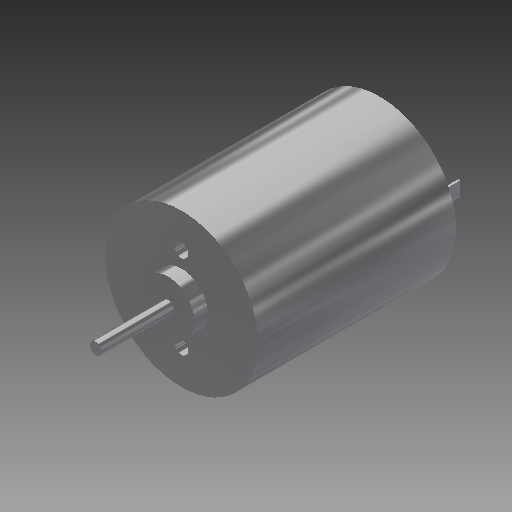
# Autodesk Inventor part: モーター(形だけ)
Saved by Autodesk Inventor 2019 (Build 230136000, 136)
## iProperties
Created: 2016-02-14
Part Number: モーター(形だけ)
Material: 一般
Document SubType Name: Modeling
Designer: 大空
Density: 2.93121 g/cm^3
Appearance: つや出し - 細かい格子状ナーリング
Mass: 75 g
Surface Area: 54.4313 cm^2
Volume: 25.5867 cm^3
Author: 大空
Autodesk Inventor part; units mm, degrees
ref_plane "YZ Plane" through (0, 0, 0) normal (1, 0, 0) x (0, 1, 0)
ref_plane "XZ Plane" through (0, 0, 0) normal (0, 1, 0) x (-1, 0, 0)
ref_plane "XY Plane" through (0, 0, 0) normal (0, 0, 1) x (1, 0, 0)
sketch "スケッチ1" plane through (0, 0, 0) normal (0, 0, 1) x (1, 0, 0)
  circle A0 centre (0, 0) radius 14.6
  circle A1 centre (0, 0) radius 5.025
  line L0 (0, 0) -> (8, 0)
  line L1 (0, 0) -> (-8, 0)
  circle A2 centre (0, 0) radius 1.15
  line L2 (-8, 0) -> (-8, -1.4)
  line L3 (-8, -1.4) -> (-8, 1.4)
  line L4 (8, 0) -> (8, -1.4)
  line L5 (8, -1.4) -> (8, 1.4)
  line L6 (8.4, -1.4) -> (8.4, 1.4)
  line L7 (-8.4, 1.4) -> (-8.4, -1.4)
  line L8 (-8.4, -1.4) -> (-8, -1.4)
  line L9 (-8.4, 1.4) -> (-8, 1.4)
  line L10 (8, -1.4) -> (8.4, -1.4)
  line L11 (8, 1.4) -> (8.4, 1.4)
  dimension "d0" = 29.2
  dimension "d1" = 10.05
  dimension "d2" = 8
  dimension "d3" = 8
  dimension "d6" = 2.3
  dimension "d21" = 1.4
  dimension "d22" = 2.8
  dimension "d23" = 1.4
  dimension "d24" = 2.8
  dimension "d25" = 0.4
  dimension "d26" = 0.4
  constraints: 24 end point, 4 vertical, 3 centre point, 3 coincident, 3 horizontal, 3 parallel, 2 point on line
  measures "d0" diameter of A0
  measures "d1" diameter of A1
  measures "d2" distance of L0.start L0.end
  measures "d3" distance of L0.start L1.end
  measures "d6" diameter of A2
  measures "d21" distance of L1.end L2.end
  measures "d22" distance of L2.end L3.end
  measures "d23" distance of L0.end L4.end
  measures "d24" distance of L4.end L5.end
  measures "d25" distance between parallel lines of L6 L4
  measures "d26" distance of L7.start L3.end
extrude "押し出し1" add sketch "スケッチ1" along normal blind 37.8 contours A0 | L0 A2 L1 A1 | L2 L8 L7 L9 L3 | A1 L1 A2 L0 | L5 L11 L6 L10 L4 | A2 L1 L0 | L0 L1 A2
extrude "押し出し2" add sketch "スケッチ1" against normal blind 2.6 contours L0 A2 L1 A1 | A1 L1 A2 L0 | A2 L1 L0 | L0 L1 A2
extrude "押し出し3" add sketch "スケッチ1" along normal blind 40.4 contours L0 A2 L1 A1 | A1 L1 A2 L0 | A2 L1 L0 | L0 L1 A2
extrude "押し出し4" add sketch "スケッチ1" along normal blind 54.2 contours A2 L1 L0 | L0 L1 A2
sketch "スケッチ2" plane through (0, 0, 37.8) normal (0, 0, 1) x (1, 0, 0)
  line L0 (0, 0) -> (0, 8)
  line L1 (0, 0) -> (0, -8)
  circle A0 centre (0, -8) radius 1.3
  circle A1 centre (0, 8) radius 1.3
  dimension "d15" = 8
  dimension "d16" = 8
  dimension "d17" = 2.6
  dimension "d18" = 2.6
  constraints: 4 end point, 2 centre point, 2 coincident
  measures "d15" distance of L0.start L0.end
  measures "d16" distance of L0.start L1.end
  measures "d17" diameter of A0
  measures "d18" diameter of A1
extrude "押し出し5" cut sketch "スケッチ2" against normal blind 15
extrude "押し出し6" add sketch "スケッチ1" against normal blind 7 contours L2 L8 L7 L9 L3 | L5 L11 L6 L10 L4
